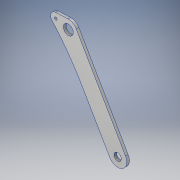
# Autodesk Inventor part: Intake Arm
Saved by Autodesk Inventor 2019.4 (Build 234330000, 330)
## iProperties
Created: 2020-01-28
Part Number: Intake Arm
Material: Aluminum 6061
Document SubType Name: Modeling
Designer: admin
Density: 2.7 g/cm^3
Appearance: Aluminum - Flat
Mass: 104.947 g
Surface Area: 187.284 cm^2
Volume: 38.8691 cm^3
Author: admin
Autodesk Inventor part; units mm, degrees
ref_plane "YZ Plane" through (0, 0, 0) normal (1, 0, 0) x (0, 1, 0)
ref_plane "XZ Plane" through (0, 0, 0) normal (0, 1, 0) x (-1, 0, 0)
ref_plane "XY Plane" through (0, 0, 0) normal (0, 0, 1) x (1, 0, 0)
sketch "Sketch1" plane through (0, 0, 0) normal (0, 0, 1) x (1, 0, 0)
  circle A0 centre (0, 0) radius 9.5
  arc A1 (-15.1554, -8.75) -> (15.1554, 8.75) centre (0, 0) ccw construction
  circle A2 centre (95, -164.5448) radius 7
  circle A3 centre (-175.4753, -121.2237) radius 88.9 construction
  circle A4 centre (95, -164.5448) radius 41.275 construction
  circle A5 centre (95, -164.5448) radius 28.5 construction
  line L0 (-263.1536, 888.7662) -> (-263.1536, -773.9924) construction
  line L1 (0, 0) -> (95, -164.5448) construction
  arc A6 (110.1554, -155.7948) -> (79.8446, -173.2948) centre (95, -164.5448) ccw construction
  line L2 (110.1554, -155.7948) -> (15.1554, 8.75)
  line L3 (79.8446, -173.2948) -> (-15.1554, -8.75)
  arc A7 (15.1554, 8.75) -> (-0.7504, 17.4839) centre (0, 0) ccw
  arc A8 (79.8446, -173.2948) -> (110.1554, -155.7948) centre (95, -164.5448) ccw
  line L4 (0, 0) -> (263.9458, 0) construction
  circle A9 centre (-24.1481, 6.4705) radius 2.5
  circle A10 centre (-24.1481, 6.4705) radius 10
  line L5 (-24.1481, 6.4705) -> (0, 0) construction
  circle A11 centre (-30, 150) radius 2.5 construction
  line L6 (-30, 150) -> (-24.1481, 6.4705) construction
  line L7 (-15.1554, -8.75) -> (-28.3706, -2.5944)
  line L8 (-24.5769, 16.4613) -> (-0.7504, 17.4839)
  arc A12 (-0.7504, 17.4839) -> (-15.1554, -8.75) centre (0, 0) ccw construction
  dimension "d0" = 19
  dimension "d1" = 35
  dimension "d4" = 14
  dimension "d5" = 177.8
  dimension "d6" = 82.55
  dimension "d7" = 57
  dimension "d8" = 190
  dimension "d9" = 35
  dimension "d10" = 60
  dimension "d11" = 5
  dimension "d12" = 20
  dimension "d13" = 25
  dimension "d14" = 135
  dimension "d15" = 5
  dimension "d16" = 150
  dimension "d17" = 30
  dimension "d18" = 143.6488
  constraints: 18 end point, 13 centre point, 12 point on circle, 8 tangent, 6 coincident, 1 horizontal, 1 vertical
  measures "d0" diameter of A0
  measures "d1" diameter of A1
  measures "d4" diameter of A2
  measures "d5" diameter of A3
  measures "d6" diameter of A4
  measures "d7" diameter of A5
  measures "d8" distance of L1.start L1.end
  measures "d9" diameter of A6
  measures "d10" angle of L1 L4
  measures "d11" diameter of A9
  measures "d12" diameter of A10
  measures "d13" distance of L5.start L1.start
  measures "d14" angle of L1 L5
  measures "d15" diameter of A11
  measures "d16" vertical distance of A0.centre L6.start
  measures "d17" horizontal distance of A0.centre L6.start
  measures "d18" distance of L6.start L5.start
extrude "Extrusion1" add sketch "Sketch1" along normal blind 5
fillet "Fillet1" radius 500 1 edges at (-15.1554, -8.75, 2.5)
body "Solid1"
